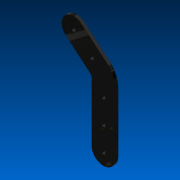
# Autodesk Inventor part: Hood Lower Bracket
Saved by Autodesk Inventor 2022 (Build 260153000, 153)
## iProperties
Created: 2022-04-17
Part Number: Hood Lower Bracket
Material: PET Plastic
Document SubType Name: Modeling
Designer: omard
Density: 1.541 g/cm^3
Appearance: Smooth - Black
Author: omard
Autodesk Inventor part; units mm, degrees
ref_plane "YZ Plane" through (0, 0, 0) normal (1, 0, 0) x (0, 1, 0)
ref_plane "XZ Plane" through (0, 0, 0) normal (0, 1, 0) x (-1, 0, 0)
ref_plane "XY Plane" through (0, 0, 0) normal (0, 0, 1) x (1, 0, 0)
sketch "Sketch1" plane through (0, 0, 0) normal (0, 0, 1) x (1, 0, 0)
  line L0 (-12.7, 25.4) -> (12.7, 25.4)
  line L1 (12.7, 25.4) -> (12.7, -25.4)
  line L2 (12.7, -25.4) -> (-12.7, -25.4)
  line L3 (-12.7, -25.4) -> (-12.7, 25.4)
  line L4 (-12.7, 25.4) -> (12.7, -25.4) construction
  line L5 (12.7, 25.4) -> (-12.7, -25.4) construction
  line L6 (-33.3465, 77.1501) -> (5.5685, 44.4965)
  line L7 (5.5685, 44.4965) -> (-10.7583, 25.039)
  line L8 (-10.7583, 25.039) -> (-49.6733, 57.6926)
  line L9 (-49.6733, 57.6926) -> (-33.3465, 77.1501)
  line L10 (-33.3465, 77.1501) -> (-10.7583, 25.039) construction
  line L11 (5.5685, 44.4965) -> (-49.6733, 57.6926) construction
  line L12 (-31.7812, 59.258) -> (-12.3236, 42.9312) construction
  line L13 (0, -12.7) -> (0, 12.7) construction
  line L14 (-12.7, -25.4) -> (12.7, -25.4)
  line L15 (12.7, -25.4) -> (12.7, -50.8)
  line L16 (12.7, -50.8) -> (-12.7, -50.8)
  line L17 (-12.7, -50.8) -> (-12.7, -25.4)
  circle A0 centre (0, -38.1) radius 12.7
  circle A1 centre (-31.7812, 59.258) radius 12.7
  line L18 (-10.7583, 25.039) -> (-185.876, 171.9802)
  arc A2 (-12.7, 25.4) -> (-13.6716, 27.4835) centre (-15.4199, 25.4) ccw
  arc A3 (12.7, 25.4) -> (5.5685, 44.4965) centre (-16.4339, 25.4) ccw
  circle A4 centre (0, -12.7) radius 12.7
  point P0 (0, 0)
  point P1 (0, 0)
  point P2 (0, 0)
  point P3 (-22.0524, 51.0946)
  point P4 (-22.0524, 51.0946)
  point P5 (-39.9446, 49.5292)
  point P6 (-12.7, -38.1)
  point P7 (12.7, -38.1)
  point P8 (-23.6178, 68.9867)
  point P9 (-10.4554, 25.4)
  point P10 (-11.1885, 25.4)
  point P11 (-41.5099, 67.4214)
  point P12 (-39.9446, 49.5292)
  point P13 (-13.6716, 27.4835)
  point P14 (-11.1885, 25.4)
  point P15 (12.7, -12.7)
  point P16 (-12.7, -12.7)
  dimension "d0" = 25.4
  dimension "d1" = 50.8
  dimension "d2" = 25.4
  dimension "d3" = 12.7
  dimension "d14" = 25.4
  constraints: 38 end point, 8 midpoint, 7 parallel, 6 tangent, 5 centre point, 4 equal length, 4 point on circle, 3 coincident, 3 perpendicular, 3 vertical alignment, 2 collinear, 2 horizontal, 1 point on line, 1 vertical, 3 other
  measures "d0" distance between parallel lines of L3 L1
  measures "d1" distance between parallel lines of L2 L0
  measures "d2" distance of L13.start L13.end
  measures "d3" distance of L13.start point (0, 0)
  measures "d14" distance of point (0, -38.1) L13.start
extrude "Extrusion1" add sketch "Sketch1" along normal blind 3.175 contours A2 L8 L0 | L0 L8 L7 L1 A4 L3 | L8 A1 L6 L7 L0 | L0 L7 L8 | A4 | L7 A3 L0 | A1
hole "Hole1" at (0, -12.7, 0) at (0, 12.7, 0) at (-12.3236, 42.9312, 0) at (-31.7812, 59.258, 0) at (0, -38.1, 0) direction (0, 0, 1) diameter 4.445 end through all
equation "\"d3\" = 0.5 * d2"
equation "\"d14\" = d2"
body "Solid1"
